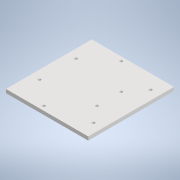
# Autodesk Inventor part: TablaBase
Saved by Autodesk Inventor 2021 (Build 250183000, 183)
## iProperties
Created: 2022-11-05
Part Number: TablaBase
Material: Genérico
Document SubType Name: Modeling
Designer: ivanm
Density: 1 g/cm^3
Appearance: Valor por defecto
Author: ivanm
Autodesk Inventor part; units mm, degrees
ref_plane "YZ Plane" through (0, 0, 0) normal (1, 0, 0) x (0, 1, 0)
ref_plane "XZ Plane" through (0, 0, 0) normal (0, 1, 0) x (-1, 0, 0)
ref_plane "XY Plane" through (0, 0, 0) normal (0, 0, 1) x (1, 0, 0)
sketch "Boceto1" plane through (0, 0, 0) normal (0, 1, 0) x (-1, 0, 0)
  line L0 (-57.0438, 614.3839) -> (-287.0438, 614.3839)
  line L1 (-287.0438, 614.3839) -> (-287.0438, 354.3839)
  line L2 (-287.0438, 354.3839) -> (-57.0438, 354.3839)
  line L3 (-57.0438, 354.3839) -> (-57.0438, 614.3839)
  circle A0 centre (-213.7553, 449.7804) radius 4 projected
  circle A1 centre (-146.7275, 368.958) radius 4 projected
  circle A2 centre (-83.2713, 432.7804) radius 4 projected
  circle A3 centre (-83.2713, 534.7804) radius 4 projected
  circle A4 centre (-146.7275, 598.6029) radius 4 projected
  circle A5 centre (-213.7553, 517.7804) radius 4 projected
  circle A6 centre (-213.7553, 449.7804) radius 4 projected
  circle A7 centre (-263.2713, 403.7804) radius 4 projected
  circle A8 centre (-263.2713, 563.7804) radius 4 projected
  circle A9 centre (-146.7275, 598.6029) radius 4
  circle A10 centre (-83.2713, 534.7804) radius 4
  circle A11 centre (-83.2713, 432.7804) radius 4
  circle A12 centre (-146.7275, 368.958) radius 4
  circle A13 centre (-213.7553, 449.7804) radius 4
  circle A14 centre (-213.7553, 517.7804) radius 4
  circle A15 centre (-263.2713, 563.7804) radius 4
  circle A16 centre (-263.2713, 403.7804) radius 4
  point P0 (0, 0)
  dimension "d0" = 230
  dimension "d1" = 260
  constraints: 8 centre point, 8 coincident, 8 concentric, 8 end point, 2 parallel, 1 horizontal, 1 perpendicular
  measures "d0" distance of L1.end L2.end
  measures "d1" distance of L0.end L1.end
extrude "Extrusión1" add sketch "Boceto1" along normal blind 10
